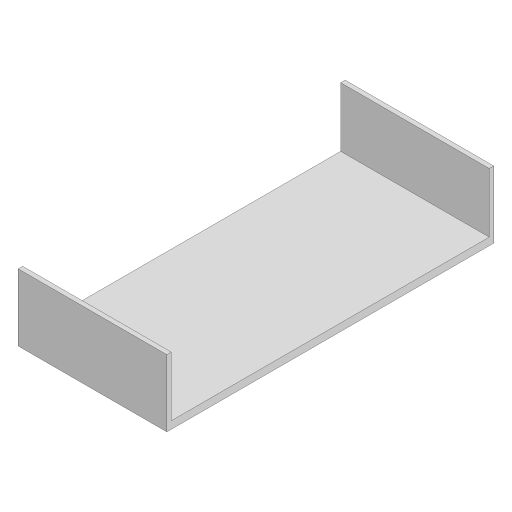
# Autodesk Inventor part: 1P10 DP3 pi holder
Saved by Autodesk Inventor 2023 (Build 270158000, 158)
## iProperties
Created: 2023-03-02
Part Number: 1P10 DP3 pi holder
Material: Generic
Document SubType Name: Modeling
Designer: Ethan Ko
Density: 1 g/cm^3
Appearance: Default
Author: Ethan Ko
Autodesk Inventor part; units mm, degrees
ref_plane "YZ Plane" through (0, 0, 0) normal (1, 0, 0) x (0, 1, 0)
ref_plane "XZ Plane" through (0, 0, 0) normal (0, 1, 0) x (-1, 0, 0)
ref_plane "XY Plane" through (0, 0, 0) normal (0, 0, 1) x (1, 0, 0)
sketch "Sketch4" plane through (0, 0, 0) normal (0, 1, 0) x (-1, 0, 0)
  line L0 (0, 0) -> (100, 0)
  line L1 (100, 0) -> (100, -220)
  line L2 (100, -220) -> (0, -220)
  line L3 (0, -220) -> (0, 0)
  dimension "d12" = 100
  dimension "d13" = 220
  constraints: 8 end point, 2 parallel, 1 horizontal, 1 perpendicular
  measures "d12" distance of L1.end L2.end
  measures "d13" distance of L0.end L1.end
extrude "Extrusion4" add sketch "Sketch4" along normal blind 5
sketch "Sketch5" plane through (0, 5, 0) normal (0, 1, 0) x (1, 0, 0)
  line L0 (-100, 220) -> (-100, 0) projected
  line L1 (-100, 0) -> (0, 0)
  line L2 (0, 0) -> (0, 3)
  line L3 (0, 3) -> (-100, 3)
  line L4 (-100, 3) -> (-100, 0)
  line L5 (-100, 220) -> (0, 220)
  line L6 (0, 220) -> (0, 217)
  line L7 (0, 217) -> (-100, 217)
  line L8 (-100, 217) -> (-100, 220)
  point P0 (0, 0)
  point P1 (-100, 217)
  dimension "d16" = 100
  dimension "d17" = 3
  dimension "d18" = 100
  dimension "d19" = 3
  constraints: 16 end point, 4 parallel, 2 horizontal, 2 perpendicular
  measures "d16" distance of L3.end L2.end
  measures "d17" distance of L2.end L1.end
  measures "d18" distance of L6.end L7.end
  measures "d19" distance of L5.end L6.end
extrude "Extrusion5" add sketch "Sketch5" along normal blind 40
body "Solid2"
